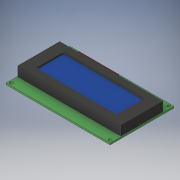
# Autodesk Inventor part: 4x20 LCD
Saved by Autodesk Inventor 2018 (Build 220112000, 112)
## iProperties
Created: 2013-10-28
Part Number: 4x20 LCD
Material: Generic
Document SubType Name: Modeling
Designer: Gabriel Smolnycki
Mass: 40.304 g
Surface Area: 149.927 cm^2
Volume: 40.304 cm^3
Density: 1 g/cm^3
Appearance: Default
Author: Gabriel Smolnycki
Sending System: SolidWorks 2017
Last Author: Gabriel Smolnycki
Last Saved: 2017-09-14
Autodesk Inventor part; units mm, degrees
ref_plane "XZ Plane" through (0, 0, 0) normal (0, 1, 0) x (-1, 0, 0)
ref_plane "XY Plane" through (0, 0, 0) normal (0, 0, 1) x (1, 0, 0)
ref_plane "Work Plane1" through (-49, 0, 0) normal (1, 0, 0) x (0, 1, 0)
sketch "Sketch1" plane through (-49, 0, 0) normal (1, 0, 0) x (0, 1, 0)
  line L0 (1.5875, -30) -> (1.5875, 30)
  line L1 (1.5875, 30) -> (0, 30)
  line L2 (0, -30) -> (0, 30)
  line L3 (1.5875, -30) -> (0, -30)
  dimension "d44" = 1.5875
  dimension "d45" = 60
  constraints: 8 end point, 2 horizontal, 2 vertical
  measures "d44" distance between parallel lines of L0 L2
  measures "d45" distance between parallel lines of L1 L3
extrude "Extrusion3" add sketch "Sketch1" along normal blind 98 draft 0
sketch "Sketch3" plane through (-49, 1.5875, 30) normal (0, 1, 0) x (1, 0, 0)
  line L0 (97.5, 50) -> (0.5, 50)
  line L1 (0.5, 50) -> (0.5, 10.5)
  line L2 (97.5, 10.5) -> (97.5, 50)
  line L3 (0.5, 10.5) -> (97.5, 10.5)
  constraints: 8 end point, 2 horizontal, 2 vertical
extrude "Extrusion2" add sketch "Sketch3" along normal blind 9
sketch "Sketch4" plane through (-49, 10.5875, 30) normal (0, 1, 0) x (1, 0, 0)
  line L0 (87, 17.25) -> (87, 43.25)
  line L1 (11, 17.25) -> (87, 17.25)
  line L2 (11, 43.25) -> (11, 17.25)
  line L3 (87, 43.25) -> (11, 43.25)
  constraints: 8 end point, 2 horizontal, 2 vertical
extrude "Extrusion1" cut sketch "Sketch4" against normal blind 1.5
hole "Hole4" at (-46.5, 1.5875, 27.5) direction (0, -1, 0) diameter 3 depth 1.5875
hole "Hole3" at (46.5, 1.5875, 27.5) direction (0, -1, 0) diameter 3 depth 1.5875
sketch "Sketch6" plane through (-49, 1.5875, 30) normal (0, 1, 0) x (1, 0, 0)
  point P0 (95.5, 2.5)
hole "Hole2" at (46.5, 1.5875, -27.5) direction (0, -1, 0) diameter 3 depth 1.5875
sketch "Sketch5" plane through (-49, 1.5875, 30) normal (0, 1, 0) x (1, 0, 0)
  point P0 (2.5, 2.5)
hole "Hole1" at (-46.5, 1.5875, -27.5) direction (0, -1, 0) diameter 3 depth 1.5875
fillet "Fillet4" radius 2 1 edges at (-38, 9.8375, -13.25)
fillet "Fillet3" radius 2 1 edges at (-38, 9.8375, 12.75)
fillet "Fillet2" radius 2 1 edges at (38, 9.8375, 12.75)
fillet "Fillet1" radius 2 1 edges at (38, 9.8375, -13.25)
sketch "Sketch9" plane through (-49, 1.5875, 30) normal (0, 1, 0) x (1, 0, 0)
  line L0 (0, 60) -> (98, 60) projected
  line L1 (9.045, 60) -> (46.854, 60)
  line L2 (46.854, 60) -> (46.854, 55.474)
  line L3 (46.854, 55.474) -> (9.045, 55.474)
  line L4 (9.045, 55.474) -> (9.045, 60)
  line L5 (0, 60) -> (0, 0) projected
  point P0 (49, 30)
  dimension "d41" = 37.809
  dimension "d42" = 4.526
  dimension "d43" = 9.045
  constraints: 8 end point, 2 parallel, 1 horizontal, 1 perpendicular, 1 point on line
  measures "d41" distance of L2.end L3.end
  measures "d42" distance of L1.end L2.end
  measures "d43" distance between parallel lines of L5 L4
extrude "Extrusion4" add sketch "Sketch9" along normal blind 0.0356
sketch "Sketch7" plane through (-49, 1.5875, 30) normal (0, 1, 0) x (1, 0, 0)
  point P0 (95.5, 57.5)
sketch "Sketch8" plane through (-49, 1.5875, 30) normal (0, 1, 0) x (1, 0, 0)
  point P0 (2.5, 57.5)
body "Solid3"
